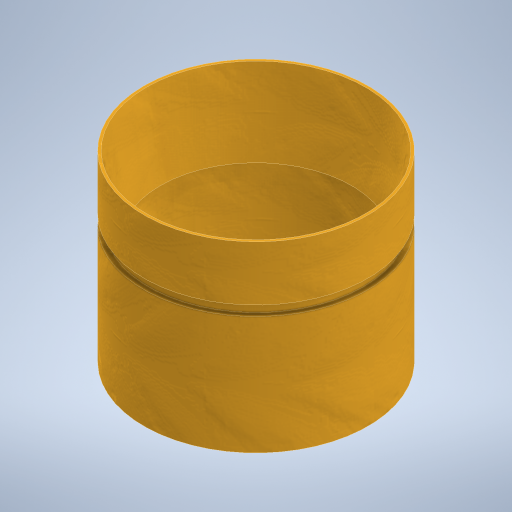
# Autodesk Inventor part: CapCone
Saved by Autodesk Inventor 2024 (Build 280153000, 153)
## iProperties
Created: 2023-09-22
Part Number: CapCone
Material: Brass, Soft Yellow, Welded
Document SubType Name: Modeling
Designer: schanen
Density: 8.5 g/cm^3
Appearance: Weld - Brass
Author: schanen
Autodesk Inventor part; units mm, degrees
ref_plane "YZ Plane" through (0, 0, 0) normal (1, 0, 0) x (0, 1, 0)
ref_plane "XZ Plane" through (0, 0, 0) normal (0, 1, 0) x (-1, 0, 0)
ref_plane "XY Plane" through (0, 0, 0) normal (0, 0, 1) x (1, 0, 0)
sketch "Sketch1" plane through (0, 0, 0) normal (0, 0, 1) x (1, 0, 0)
  line L0 (-19.225, -30) -> (-22.225, -30) construction
  line L1 (-22.225, -30) -> (-22.225, -20) construction
  line L2 (-22.225, -20) -> (-19.225, -20) construction
  line L3 (-19.225, -20) -> (-19.225, -30) construction
  line L4 (-22, 36.7378) -> (-19.225, 21)
  line L5 (-22.5, 0) -> (-22.5, 23.7378)
  line L6 (-22.5, 23.7378) -> (-21.5, 23.7378)
  line L7 (-21.5, 23.7378) -> (-21.5, 25.7378)
  line L8 (-21.5, 25.7378) -> (-22.5, 25.7378)
  line L9 (-22.5, 25.7378) -> (-22.5, 36.7378)
  line L10 (-22, 36.7378) -> (-22.5, 36.7378)
  line L11 (0, -43.3476) -> (0, 50.0854) projected
  line L12 (-19.225, -20) -> (-20.225, -20) construction
  line L13 (-20.225, -20) -> (-20.225, 0) construction
  line L14 (-20.225, 0) -> (-19.225, 0) construction
  line L15 (-19.225, 0) -> (-19.225, -20) construction
  line L16 (-22.5, 0) -> (-20.225, 0)
  line L17 (-20.225, 0) -> (-20.225, 21)
  line L18 (-20.225, 21) -> (-19.225, 21)
  point P0 (0, 0)
  dimension "d0" = 10
  dimension "d1" = 22.225
  dimension "d3" = 3
  dimension "d5" = 11
  dimension "d6" = 2
  dimension "d7" = 22.5
  dimension "d10" = 21
  dimension "d12" = 1
  dimension "d16" = 20
  dimension "d17" = 1
  dimension "d18" = 0.5
  dimension "d19" = 10
  constraints: 36 end point, 6 perpendicular, 5 horizontal, 4 parallel, 2 horizontal alignment, 2 point on line, 1 coincident, 1 vertical, 1 vertical alignment
  measures "d0" distance of L0.end L1.end
  measures "d1" distance from line of point (0, 0) L1
  measures "d3" distance of L0.end L0.start
  measures "d5" distance of L8.end L9.end
  measures "d6" distance of L6.end L7.end
  measures "d7" distance from line of point (0, 0) L5
  measures "d10" vertical distance of L5.start L4.end
  measures "d12" distance of L5.end L6.end
  measures "d16" distance of L12.end L13.end
  measures "d17" distance between parallel lines of L15 L13
  measures "d18" distance of L4.start L9.end
  measures "d19" angle of L4 L9
revolve "Revolution1" add sketch "Sketch1" angle 360 about axis through (0, -10, 0) along (0, 1, 0)
body "Solid1"
